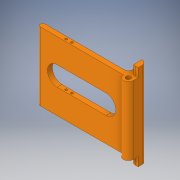
# Autodesk Inventor part: Bottom-Lip
Saved by Autodesk Inventor 2018.3 (Build 223284000, 284)
## iProperties
Created: 2018-05-20
Part Number: Bottom-Lip
Material: Generisch
Document SubType Name: Modeling
Designer: JochenAlt
Density: 1 g/cm^3
Appearance: Orange
Author: JochenAlt
Autodesk Inventor part; units mm, degrees
ref_plane "YZ Plane" through (0, 0, 0) normal (1, 0, 0) x (0, 1, 0)
ref_plane "XZ Plane" through (0, 0, 0) normal (0, 1, 0) x (-1, 0, 0)
ref_plane "XY Plane" through (0, 0, 0) normal (0, 0, 1) x (1, 0, 0)
sketch "Skizze1" plane through (0, 0, 0) normal (0, 0, 1) x (1, 0, 0)
  line L0 (0, 9.4989) -> (0, -4.4998) construction
  line L1 (-56.1636, 0) -> (12.8813, 0) construction
  circle A0 centre (0, 0) radius 2.5
  arc A1 (-45, 2.5) -> (-45, 0) centre (-45, 1.25) ccw
  line L2 (-45, 2.5) -> (-4.5, 2.5)
  line L3 (-45, 0) -> (-2.5, 0)
  circle A2 centre (0, 0) radius 1.2
  circle A3 centre (-45, 1.2) radius 1.3
  line L4 (0, 2.5) -> (0, 6.9813)
  arc A4 (2.5, 4.4813) -> (0, 6.9813) centre (0, 4.4813) ccw
  line L5 (2.5, 2.5) -> (2.5, 0)
  line L6 (1.0198, 2.5) -> (2.5, 2.5)
  line L7 (2.5, 2.5) -> (2.5, 4.4813)
  arc A5 (0, 6.9813) -> (-2.5, 4.4813) centre (0, 4.4813) ccw
  line L8 (-2.5, 4.4813) -> (-2.5, 4.5)
  arc A6 (-4.5, 2.5) -> (-2.5, 4.5) centre (-4.5, 4.5) ccw
  arc A7 (1.0198, 2.5) -> (0, 2.7) centre (0, 0) ccw
  circle A8 centre (-33, 1.2) radius 0.6
  circle A9 centre (-30, 1.2) radius 0.6
  line L9 (-45, 1.2) -> (0, 1.2) construction
  point P0 (-2.5, 0)
  dimension "d3" = 2.4
  dimension "d0" = 5
  dimension "d1" = 2.5
  dimension "d6" = 45
  dimension "d21" = 2
  dimension "d22" = 0.2
  dimension "d23" = 1.2
  dimension "d24" = 3
  dimension "d25" = 30
  constraints: 16 end point, 14 point on circle, 9 tangent, 8 centre point, 6 point on line, 3 coincident, 3 equal radius, 3 horizontal, 2 parallel, 2 vertical alignment, 1 concentric, 1 line through centre, 1 vertical, 4 other
  measures "d0" diameter of A0
  measures "d1" diameter of A1
  measures "d6" distance from line of L0 A1.centre
  measures "d21" radius of A6
  measures "d22" radial gap between concentric circles of A7 A0
  measures "d23" diameter of A8
  measures "d24" distance of A9.centre A8.centre
  measures "d25" distance from line of L0 A9.centre
extrude "Extrusion1" add sketch "Skizze1" along normal mid plane 35 contours A0 | A0 L4 A7 L6 L5 | A0 L3 A3 L2 A6 A5 L4 | L3 A1 A3 picked at (-45.3896, 1.1022)
extrude "Extrusion6" add sketch "Skizze1" along normal mid plane 44 contours L6 A7 L4 A4 L7
sketch "Skizze2" plane through (-45, 0, 17.5) normal (0, -1, 0) x (1, 0, 0)
  line L0 (8.5763, -17.4438) -> (33.5763, -17.4438) construction
  line L1 (8.5763, -22.4438) -> (33.5763, -22.4438)
  line L2 (33.5763, -12.4438) -> (8.5763, -12.4438)
  arc A0 (8.5763, -12.4438) -> (8.5763, -22.4438) centre (8.5763, -17.4438) ccw
  arc A1 (33.5763, -22.4438) -> (33.5763, -12.4438) centre (33.5763, -17.4438) ccw
  point P0 (45, -17.5)
  point P1 (21.0763, -17.4438)
  dimension "d26" = 10
  dimension "d27" = 25
  constraints: 8 end point, 4 point on circle, 4 tangent, 2 centre point, 1 horizontal, 1 midpoint, 1 parallel
  measures "d26" diameter of A1
  measures "d27" distance of L0.end L0.start
extrude "Extrusion7" cut sketch "Skizze2" against normal through all
